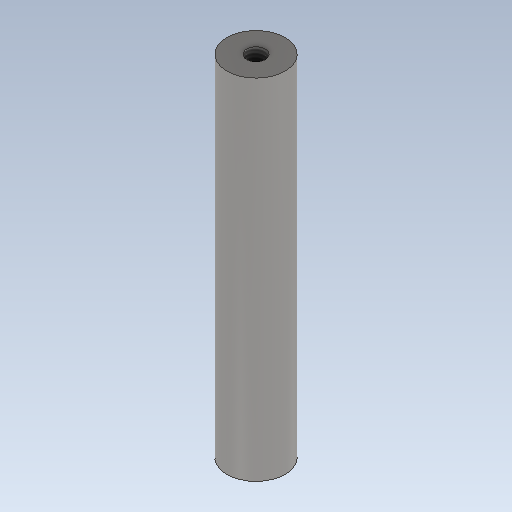
# Autodesk Inventor part: Pieza1
Saved by Autodesk Inventor 2020.3 (Build 243373000, 373)
## iProperties
Created: 2020-11-14
Part Number: Pieza1
Material: Acero inoxidable
Document SubType Name: Modeling
Designer: codig
Density: 8 g/cm^3
Appearance: Semipulido
Author: codig
Autodesk Inventor part; units mm, degrees
ref_plane "YZ Plane" through (0, 0, 0) normal (1, 0, 0) x (0, 1, 0)
ref_plane "XZ Plane" through (0, 0, 0) normal (0, 1, 0) x (-1, 0, 0)
ref_plane "XY Plane" through (0, 0, 0) normal (0, 0, 1) x (1, 0, 0)
sketch "Boceto1" plane through (0, 0, 0) normal (0, 1, 0) x (-1, 0, 0)
  circle A0 centre (0, 0) radius 12.5
  constraints: 1 centre point, 1 coincident
extrude "Extrusión1" add sketch "Boceto1" along normal blind 150
sketch "Boceto2" plane through (0, 150, 0) normal (0, 1, 0) x (1, 0, 0)
  circle A0 centre (0, 0) radius 12.5 projected
  circle A1 centre (0, 0) radius 4
  constraints: 1 centre point, 1 coincident
hole "Agujero1" at (0, 150, 0) direction (0, -1, 0) diameter 8 end through all
thread "Rosca1" size "3/8-16 UNC" class "1B" standard "ANSI Unified Screw Threads" full length
